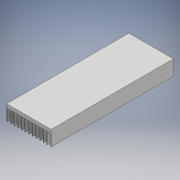
# Autodesk Inventor part: heat sink
Saved by Autodesk Inventor 2018 (Build 220112000, 112)
## iProperties
Created: 2018-06-04
Part Number: heat sink
Material: Generic
Document SubType Name: Modeling
Designer: John Viljoen
Density: 1 g/cm^3
Appearance: Default
Author: John Viljoen
Autodesk Inventor part; units mm, degrees
ref_plane "YZ Plane" through (0, 0, 0) normal (1, 0, 0) x (0, 1, 0)
ref_plane "XZ Plane" through (0, 0, 0) normal (0, 1, 0) x (-1, 0, 0)
ref_plane "XY Plane" through (0, 0, 0) normal (0, 0, 1) x (1, 0, 0)
sketch "Sketch1" plane through (0, 0, 0) normal (0, 0, 1) x (1, 0, 0)
  line L0 (0, 0) -> (97.3, 0)
  line L1 (97.3, 0) -> (97.3, 267)
  line L2 (97.3, 267) -> (0, 267)
  line L3 (0, 267) -> (0, 0)
  dimension "d0" = 97.3
  dimension "d1" = 267
  constraints: 8 end point, 2 perpendicular, 1 horizontal, 1 vertical
  measures "d0" distance of L0.start L0.end
  measures "d1" distance of L0.end L1.end
extrude "Extrusion1" add sketch "Sketch1" along normal blind 7.8
sketch "Sketch2" plane through (0, 0, 0) normal (0, -1, 0) x (1, 0, 0)
  line L0 (0, 0) -> (97.3, 0) projected
  line L1 (0, 0) -> (1.8, 0)
  line L2 (1.8, 0) -> (1.8, -25.2)
  line L3 (1.8, -25.2) -> (0, -25.2)
  line L4 (0, -25.2) -> (0, 0)
  line L5 (9.7583, 0) -> (9.7583, -25.2)
  line L6 (7.9583, 0) -> (9.7583, 0)
  line L7 (7.9583, -25.2) -> (7.9583, 0)
  line L8 (9.7583, -25.2) -> (7.9583, -25.2)
  line L9 (17.7167, 0) -> (17.7167, -25.2)
  line L10 (15.9167, 0) -> (17.7167, 0)
  line L11 (15.9167, -25.2) -> (15.9167, 0)
  line L12 (17.7167, -25.2) -> (15.9167, -25.2)
  line L13 (25.675, 0) -> (25.675, -25.2)
  line L14 (23.875, 0) -> (25.675, 0)
  line L15 (23.875, -25.2) -> (23.875, 0)
  line L16 (25.675, -25.2) -> (23.875, -25.2)
  line L17 (33.6333, 0) -> (33.6333, -25.2)
  line L18 (31.8333, 0) -> (33.6333, 0)
  line L19 (31.8333, -25.2) -> (31.8333, 0)
  line L20 (33.6333, -25.2) -> (31.8333, -25.2)
  line L21 (41.5917, 0) -> (41.5917, -25.2)
  line L22 (39.7917, 0) -> (41.5917, 0)
  line L23 (39.7917, -25.2) -> (39.7917, 0)
  line L24 (41.5917, -25.2) -> (39.7917, -25.2)
  line L25 (49.55, 0) -> (49.55, -25.2)
  line L26 (47.75, 0) -> (49.55, 0)
  line L27 (47.75, -25.2) -> (47.75, 0)
  line L28 (49.55, -25.2) -> (47.75, -25.2)
  line L29 (57.5083, 0) -> (57.5083, -25.2)
  line L30 (55.7083, 0) -> (57.5083, 0)
  line L31 (55.7083, -25.2) -> (55.7083, 0)
  line L32 (57.5083, -25.2) -> (55.7083, -25.2)
  line L33 (65.4667, 0) -> (65.4667, -25.2)
  line L34 (63.6667, 0) -> (65.4667, 0)
  line L35 (63.6667, -25.2) -> (63.6667, 0)
  line L36 (65.4667, -25.2) -> (63.6667, -25.2)
  line L37 (73.425, 0) -> (73.425, -25.2)
  line L38 (71.625, 0) -> (73.425, 0)
  line L39 (71.625, -25.2) -> (71.625, 0)
  line L40 (73.425, -25.2) -> (71.625, -25.2)
  line L41 (81.3833, 0) -> (81.3833, -25.2)
  line L42 (79.5833, 0) -> (81.3833, 0)
  line L43 (79.5833, -25.2) -> (79.5833, 0)
  line L44 (81.3833, -25.2) -> (79.5833, -25.2)
  line L45 (89.3417, 0) -> (89.3417, -25.2)
  line L46 (87.5417, 0) -> (89.3417, 0)
  line L47 (87.5417, -25.2) -> (87.5417, 0)
  line L48 (89.3417, -25.2) -> (87.5417, -25.2)
  line L49 (97.3, 0) -> (97.3, -25.2)
  line L50 (95.5, 0) -> (97.3, 0)
  line L51 (95.5, -25.2) -> (95.5, 0)
  line L52 (97.3, -25.2) -> (95.5, -25.2)
  dimension "d4" = 1.8
  dimension "d5" = 25.2
  dimension "d8" = 7.9583
  constraints: 104 end point, 2 horizontal, 2 parallel, 1 perpendicular, 96 other
  measures "d4" distance of L2.end L3.end
  measures "d5" distance of L1.end L2.end
  measures "d8" distance of L1.end L5.start
extrude "Extrusion2" add sketch "Sketch2" against normal up to surface (267 mm away)
body "Solid1"
